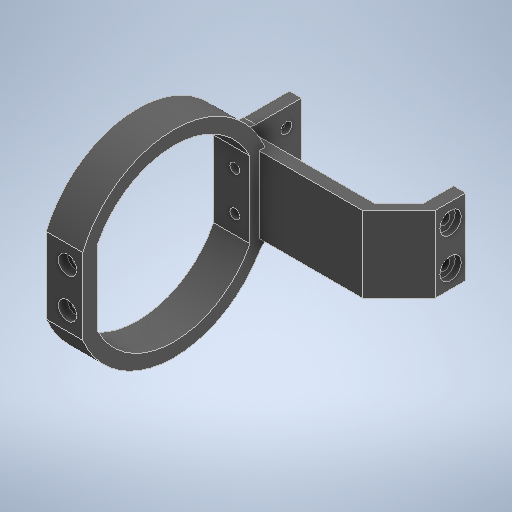
# Autodesk Inventor part: volume_connection
Saved by Autodesk Inventor 2026.1 (Build 301233020, 233B)
## iProperties
Created: 2026-02-03
Part Number: volume_connection
Material: 一般
Document SubType Name: Modeling
Designer: hibik
Density: 1 g/cm^3
Appearance: 既定
Author: hibik
Autodesk Inventor part; units mm, degrees
ref_plane "YZ Plane" through (0, 0, 0) normal (1, 0, 0) x (0, 1, 0)
ref_plane "XZ Plane" through (0, 0, 0) normal (0, 1, 0) x (-1, 0, 0)
ref_plane "XY Plane" through (0, 0, 0) normal (0, 0, 1) x (1, 0, 0)
sketch "スケッチ1" plane through (0, 0, 0) normal (0, 1, 0) x (-1, 0, 0)
  line L0 (-29, -10) -> (-25, -10)
  line L1 (-25, -10) -> (-25, 0)
  line L2 (-25, 0) -> (-29, 0)
  line L3 (-29, 0) -> (-29, -10)
  line L4 (25, -10) -> (29, -10)
  line L5 (29, -10) -> (29, 0)
  line L6 (29, 0) -> (25, 0)
  line L7 (25, 0) -> (25, -10)
  line L8 (25, 0) -> (-25, 0)
  line L9 (29, 0) -> (25, 0)
  line L10 (25, 0) -> (25, 12)
  line L11 (25, 12) -> (29, 12)
  line L12 (29, 12) -> (29, 0)
  line L13 (29, 12) -> (-17, 12)
  line L14 (-17, 12) -> (-17, 8)
  line L15 (-17, 8) -> (29, 8)
  line L16 (29, 8) -> (29, 12)
  line L17 (-17, 12) -> (-29, 0)
  line L18 (-25, 0) -> (-17, 8)
  point P0 (0, 0)
  point P1 (0, 0)
  point P2 (25, 8)
  dimension "d0" = 50
  dimension "d1" = 10
  dimension "d2" = 4
  dimension "d3" = 45
  dimension "d4" = 8
  constraints: 38 end point, 9 parallel, 5 horizontal, 4 perpendicular, 2 collinear, 2 equal length, 1 coincident, 1 midpoint
  measures "d0" distance between parallel lines of L1 L7
  measures "d1" distance of L4.end L5.end
  measures "d2" distance of L5.end L6.end
  measures "d3" angle of L8 L18
  measures "d4" distance between parallel lines of L8 L15
extrude "押し出し1" add sketch "スケッチ1" along normal blind 25 contours L3 L2 L1 L0 | L17 L14 L18 L2 | L13 L10 L15 L14 | L10 L15 L12 L6 | L6 L5 L4 L7 | L11 L12 L15 L10
sketch "スケッチ2" plane through (17, 0, 8) normal (0, 0, -1) x (-1, 0, 0)
  circle A0 centre (39, 19) radius 1.6
  circle A1 centre (39, 6) radius 1.6
  line L0 (0, 0) -> (42, 0) projected
  line L1 (0, 25) -> (42, 25) projected
  line L2 (42, 0) -> (42, 25) projected
  point P0 (17, 0)
  dimension "d7" = 3.2
  dimension "d8" = 3.2
  dimension "d9" = 6
  dimension "d10" = 6
  dimension "d11" = 3
  constraints: 2 centre point, 1 vertical alignment
  measures "d7" diameter of A0
  measures "d8" diameter of A1
  measures "d9" distance from line of A1.centre L0
  measures "d10" distance from line of L1 A0.centre
  measures "d11" distance from line of L2 A0.centre
extrude "押し出し2" cut sketch "スケッチ2" against normal through all
sketch "スケッチ3" plane through (17, 0, 8) normal (0, 0, -1) x (-1, 0, 0)
  circle A0 centre (39, 19) radius 1.6 projected
  circle A1 centre (39, 6) radius 1.6 projected
  circle A2 centre (39, 19) radius 3
  circle A3 centre (39, 6) radius 3
  point P0 (17, 0)
  dimension "d14" = 6
  dimension "d15" = 6
  constraints: 2 centre point, 2 coincident
  measures "d14" diameter of A2
  measures "d15" diameter of A3
extrude "押し出し3" cut sketch "スケッチ3" against normal blind 2 contours A0 | A1 | A2 | A3
sketch "スケッチ4" plane through (29, 0, 0) normal (1, 0, 0) x (0, 0, -1)
  circle A0 centre (5, 19) radius 1.75
  circle A1 centre (5, 6) radius 1.75
  line L0 (0, 0) -> (0, 25) projected
  line L1 (0, 12.5) -> (10, 12.5)
  line L2 (10, 0) -> (10, 25) projected
  line L3 (0, 25) -> (10, 25) projected
  point P0 (5, 12.5)
  dimension "d18" = 6
  dimension "d19" = 3.5
  constraints: 3 midpoint, 2 centre point, 2 end point, 1 horizontal, 1 vertical alignment, 1 other
  measures "d18" distance from line of L3 A0.centre
  measures "d19" diameter of A0
extrude "押し出し4" cut sketch "スケッチ4" against normal blind 4 contours A0 | A1
sketch "スケッチ5" plane through (29, 0, 0) normal (1, 0, 0) x (0, 0, -1)
  circle A0 centre (5, 19) radius 1.75 projected
  circle A1 centre (5, 6) radius 1.75 projected
  circle A2 centre (5, 19) radius 3.5
  circle A3 centre (5, 6) radius 3.5
  point P0 (0, 0)
  dimension "d22" = 7
  dimension "d23" = 7
  constraints: 2 centre point, 2 coincident
  measures "d22" diameter of A2
  measures "d23" diameter of A3
extrude "押し出し5" cut sketch "スケッチ5" against normal blind 2 contours A0 | A1 | A2 | A3
ref_plane "作業平面1" through (0, 0, 0) normal (1, 0, 0) x (0, 0, -1)
mirror "ミラー1" about plane through (0, 0, 0) normal (1, 0, 0) of "押し出し4", "押し出し5"
sketch "スケッチ6" plane through (-29, 0, 12) normal (0, 0, 1) x (1, 0, 0)
  circle A0 centre (7, 6) radius 1.6 projected
  circle A1 centre (7, 19) radius 1.6 projected
  line L0 (0, 0) -> (46, 0) projected
  line L1 (46, 0) -> (46, 25) projected
  line L2 (0, 25) -> (46, 25) projected
  line L3 (0, 0) -> (0, 25) projected
  line L4 (12, 0) -> (2, 0)
  line L5 (2, 0) -> (2, 25)
  line L6 (2, 25) -> (12, 25)
  line L7 (12, 25) -> (12, 0)
  line L8 (0, 0) -> (46, 0) projected
  point P0 (29, 0)
  point P1 (7, 0)
  point P2 (12, 0)
  point P3 (12, 25)
  dimension "d26" = 10
  dimension "d27" = 25
  constraints: 8 end point, 2 parallel, 1 horizontal, 1 midpoint, 1 perpendicular, 1 point on line, 1 vertical alignment
  measures "d26" distance of L5.end L6.end
  measures "d27" distance of L4.end L5.end
extrude "押し出し6" add sketch "スケッチ6" along normal blind 3 contours L5 L2 L7 L0
ref_plane "作業平面2" through (-29, 0, 65) normal (0, 0, 1) x (1, 0, 0)
sketch "スケッチ7" plane through (-29, 0, 65) normal (0, 0, 1) x (1, 0, 0)
  line L0 (12, 25) -> (2, 25) projected
  line L1 (2, 25) -> (2, 0) projected
  line L2 (2, 0) -> (12, 0) projected
  line L3 (12, 0) -> (12, 25) projected
  circle A0 centre (7, 6) radius 1.6 projected
  circle A1 centre (7, 19) radius 1.6 projected
  point P0 (29, 0)
extrude "押し出し7" add sketch "スケッチ7" along normal blind 2
sketch "スケッチ8" plane through (-29, 0, 67) normal (0, 0, 1) x (1, 0, 0)
  line L0 (2, 25) -> (2, 0) projected
  line L1 (2, 0) -> (12, 0) projected
  line L2 (12, 0) -> (12, 25) projected
  line L3 (12, 25) -> (2, 25) projected
  circle A0 centre (7, 6) radius 1.6 projected
  circle A1 centre (7, 19) radius 1.6 projected
  circle A2 centre (7, 19) radius 3 projected
  circle A3 centre (7, 6) radius 3 projected
  point P0 (29, 0)
  point P1 (4, 19)
  point P2 (4, 6)
  constraints: 2 horizontal alignment
extrude "押し出し8" add sketch "スケッチ8" along normal blind 3 contours L3 L2 L1 L0
sketch "スケッチ9" plane through (-27, 0, 65) normal (-1, 0, 0) x (0, 0, 1)
  line L0 (0, 25) -> (5, 25) projected
  circle A0 centre (-25, 12.5) radius 27.9508
  circle A1 centre (-25, 12.5) radius 32.5
  line L1 (0, 25) -> (0, 0) projected
  line L2 (-53, 25) -> (-50, 25) projected
  line L3 (-75, 25) -> (-53, 25) projected
  line L4 (-50, 25) -> (-55, 25)
  line L5 (5, 25) -> (0, 25)
  line L6 (-50, 0) -> (-55, 0)
  line L7 (0, 0) -> (5, 0)
  point P0 (-65, 0)
  point P1 (0, 12.5)
  point P2 (0, 12.5)
  point P3 (-50, 0)
  dimension "d35" = 25
  constraints: 8 end point, 7 point on circle, 3 horizontal, 2 centre point, 2 midpoint, 2 point on line, 1 coincident, 1 horizontal alignment
  measures "d35" distance of point (0, 12.5) A0.centre
extrude "押し出し9" add sketch "スケッチ9" against normal up to surface (10 mm away) contours A0 L2 L3 A1 L0 | L7 A1 L6 A0
sketch "スケッチ10" plane through (-27, 0, 12) normal (-1, 0, 0) x (0, 0, 1)
  line L0 (53, 25) -> (53, 0) projected
  arc A0 (3, 0) -> (53, 0) centre (28, 12.5) ccw projected
  line L1 (3, 25) -> (3, 0) projected
  arc A1 (53, 25) -> (3, 25) centre (28, 12.5) ccw projected
  arc A2 (58, 25) -> (-2, 25) centre (28, 12.5) ccw projected
  line L2 (0, 25) -> (-2, 25) projected
  line L3 (0, 0) -> (0, 25) projected
  line L4 (-2, 0) -> (0, 0) projected
  arc A3 (-2, 0) -> (58, 0) centre (28, 12.5) ccw projected
  line L5 (58, 25) -> (58, 0) projected
  point P0 (-12, 0)
extrude "押し出し10" add sketch "スケッチ10" along normal up to surface (2 mm away)
fillet "フィレット1" radius 8 2 edges at (-23, 25, 10) (-23, 0, 10)
equation "\"d10\" = d9"
